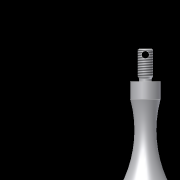
# Autodesk Inventor part: Glocke03
Saved by Autodesk Inventor 2013 (Build 170138000, 138)
## iProperties
Created: 2005-03-10
Part Number: Glocke03
Document SubType Name: Modeling
Designer: acad
Manufacturer: Standard
Standards Organization: Custom
Material: Allgemein
Density: 1 g/cm^3
Author: acad
Autodesk Inventor part; units mm, degrees
ref_plane "YZ Plane" through (0, 0, 0) normal (1, 0, 0) x (0, 1, 0)
ref_plane "XZ Plane" through (0, 0, 0) normal (0, 1, 0) x (-1, 0, 0)
sketch "Skizze1" plane through (0, 0, 0) normal (0, 0, 1) x (1, 0, 0)
  line L0 (51.4579, -0.3839) -> (-27.7559, -0.3839)
  arc A0 (51.4579, -0.3839) -> (33.7598, 9.9902) centre (39.5684, -0.3839) ccw
  arc A1 (-1.5421, 5.6161) -> (33.7598, 9.9902) centre (10.745, 51.0944) ccw
  line L1 (-1.5421, 5.6161) -> (-8.5421, 5.6161)
  line L2 (-8.5421, 5.6161) -> (-8.5421, -0.3839)
  line L3 (-8.5421, 2.1161) -> (-9.6248, 2.1161)
  line L4 (-9.6248, 2.1161) -> (-10.5421, 2.6161)
  line L5 (-10.5421, 2.6161) -> (-21.5421, 2.6161)
  line L6 (-21.5421, 2.6161) -> (-21.5421, -0.3839)
  dimension "d0" = 60
  dimension "d1" = 7
  dimension "d2" = 3
  dimension "d3" = 2.5
  dimension "d4" = 11
  dimension "d5" = 13
  dimension "d6" = 6
  constraints: 14 end point, 4 point on circle, 4 point on line, 3 perpendicular, 2 centre point, 2 parallel, 1 horizontal, 1 tangent
  measures "d0" distance of L0.start L2.end
  measures "d1" distance of L1.start L1.end
  measures "d2" distance of L5.end L6.end
  measures "d3" distance of L2.end L3.start
  measures "d4" distance of L4.end L5.end
  measures "d5" distance of L6.end L2.end
  measures "d6" distance of L2.end L1.end
revolve "Drehung1" add sketch "Skizze1" angle 360 about axis through (51.4579, -0.3839, 0) along (-1, 0, 0)
chamfer "Fase1" distance 0.5 angle 45 1 edges at (-21.5421, -3.3839, 0)
thread "Gewinde1" size "M6x1" class "6g" standard "ANSI Metrisches M Profil" full length
ref_plane "Arbeitsebene1" through (-16.0421, -0.3839, 3) normal (0, 0, 1) x (1, 0, 0)
sketch "Skizze2" plane through (-16.0421, -0.3839, 3) normal (0, 0, 1) x (1, 0, 0)
  line L0 (-5, 3) -> (-5, -3) projected
  line L1 (5.5, -3) -> (5.5, 3) projected
  line L2 (-5, 3) -> (-5, -3) projected
  line L3 (-5, 3) -> (5.5, 3) projected
  line L4 (-5, -3) -> (5.5, -3) projected
  line L5 (-5.5, -2.5) -> (-5.5, 2.5) projected
  point P0 (-3.1, 0)
  dimension "d14" = 3
  dimension "d15" = 2.4
  measures "d14" distance from line of L3 point (-3.1, 0)
  measures "d15" distance from line of L5 point (-3.1, 0)
hole "Bohrung1" at (-19.1421, -0.3839, 3) direction (0, 0, -1) diameter 3 end through all
